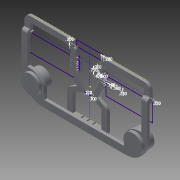
# Autodesk Inventor part: alignment_tool
Saved by Autodesk Inventor 2015 SP1 (Build 190203100, 203)
## iProperties
Created: 2015-09-17
Part Number: alignment_tool
Material: Generic
Document SubType Name: Modeling
Designer: tankadmin
Density: 1 g/cm^3
Appearance: Default
Author: tankadmin
Autodesk Inventor part; units mm, degrees
ref_plane "YZ Plane" through (0, 0, 0) normal (1, 0, 0) x (0, 1, 0)
ref_plane "XZ Plane" through (0, 0, 0) normal (0, 1, 0) x (-1, 0, 0)
ref_plane "XY Plane" through (0, 0, 0) normal (0, 0, 1) x (1, 0, 0)
sketch "Sketch1" plane through (0, 0, 0) normal (0, 0, 1) x (1, 0, 0)
  line L0 (-44.45, -76.2) -> (44.45, -76.2)
  line L1 (44.45, -76.2) -> (44.45, -19.05)
  line L2 (44.45, -19.05) -> (22.614, -6.964)
  line L3 (22.614, -6.964) -> (37.9893, 20.8148)
  line L4 (37.9893, 20.8148) -> (75.5958, 0)
  line L5 (75.5958, 0) -> (139.7, 0)
  line L6 (139.7, 0) -> (139.7, 76.2)
  line L7 (139.7, 76.2) -> (-139.7, 76.2)
  line L8 (-139.7, 76.2) -> (-139.7, 0)
  line L9 (-139.7, 0) -> (-75.5958, 0)
  line L10 (-75.5958, 0) -> (-37.9893, 20.8148)
  line L11 (-37.9893, 20.8148) -> (-22.614, -6.964)
  line L12 (-22.614, -6.964) -> (-44.45, -19.05)
  line L13 (-44.45, -19.05) -> (-44.45, -76.2)
  line L14 (0, -76.2) -> (0, 76.2) construction
  line L15 (-127, 63.5) -> (127, 63.5)
  line L16 (127, 63.5) -> (127, 12.7)
  line L17 (127, 12.7) -> (73.6309, 12.7)
  line L18 (73.6309, 12.7) -> (34.0201, 34.6241)
  line L19 (34.0201, 34.6241) -> (8.8047, -10.9331)
  line L20 (8.8047, -10.9331) -> (31.75, -23.6331)
  line L21 (31.75, -23.6331) -> (31.75, -63.5)
  line L22 (31.75, -63.5) -> (-31.75, -63.5)
  line L23 (-31.75, -63.5) -> (-31.75, -23.6331)
  line L24 (-31.75, -23.6331) -> (-8.8047, -10.9331)
  line L25 (-8.8047, -10.9331) -> (-34.0201, 34.6241)
  line L26 (-34.0201, 34.6241) -> (-73.6309, 12.7)
  line L27 (-73.6309, 12.7) -> (-127, 12.7)
  line L28 (-127, 12.7) -> (-127, 63.5)
  line L29 (139.7, 38.1) -> (-139.7, 38.1) construction
  line L30 (139.7, 19.05) -> (-139.7, 19.05) construction
  point P0 (0, 0)
  point P1 (0, 0)
  point P2 (0, 19.05)
  point P3 (25.4, 19.05)
  point P4 (-25.4, 19.05)
  dimension "d2" = 88.9
  dimension "d4" = 279.4
  dimension "d8" = 76.2
  dimension "d10" = 12.7
  dimension "d11" = 10.16
  dimension "d12" = 10.16
  dimension "d13" = 10.16
  dimension "d14" = 12.7
  dimension "d15" = 10.16
  dimension "d16" = 10.16
  dimension "d17" = 10.16
  dimension "d18" = 12.7
  dimension "d19" = 12.7
  dimension "d97" = 19.05
  dimension "d98" = 25.4
  dimension "d99" = 31.75
  dimension "d100" = 25.4
  dimension "d101" = 31.75
  dimension "d102" = 12.7
  dimension "d151" = 31.75
  dimension "d152" = 57.15
  dimension "d153" = 76.2
  constraints: 62 end point, 17 perpendicular, 8 point on line, 6 midpoint, 2 equal length, 1 coincident, 1 horizontal, 4 other
  measures "d2" distance between parallel lines of L1 L13
  measures "d4" distance between parallel lines of L6 L8
  measures "d8" distance between parallel lines of L0 L9
  measures "d10" distance between parallel lines of L22 L0
  measures "d11" distance between parallel lines of L24 L12
  measures "d12" distance between parallel lines of L25 L11
  measures "d13" distance between parallel lines of L10 L26
  measures "d14" distance between parallel lines of L9 L27
  measures "d15" distance between parallel lines of L2 L20
  measures "d16" distance between parallel lines of L3 L19
  measures "d17" distance between parallel lines of L4 L18
  measures "d18" distance between parallel lines of L5 L17
  measures "d19" distance between parallel lines of L6 L16
  measures "d97" distance between parallel lines of L30 L29
  measures "d98" distance of point (0, 19.05) point (25.4, 19.05)
  measures "d99" distance between parallel lines of L2 L4
  measures "d100" distance of point (-25.4, 19.05) point (0, 19.05)
  measures "d101" distance between parallel lines of L10 L12
  measures "d102" vertical distance of L19.end L20.end
  measures "d151" distance from line of L17 L1.end
  measures "d152" distance from line of L1.end L29
  measures "d153" distance between parallel lines of L5 L7
extrude "Extrusion1" add sketch "Sketch1" along normal blind 6.35
sketch "Sketch2" plane through (0, 0, 6.35) normal (0, 0, 1) x (1, 0, 0)
  line L0 (31.75, -63.5) -> (-31.75, -63.5) construction
  line L1 (139.7, 50.8) -> (139.7, -78.74)
  line L2 (139.7, -78.74) -> (-139.7, -78.74)
  line L3 (-139.7, -78.74) -> (-139.7, 50.8)
  circle A0 centre (-114.3, -43.18) radius 13.081
  line L4 (0, -78.74) -> (0, 75.1889) construction
  line L5 (-139.7, 45.72) -> (139.7, 45.72) construction
  circle A1 centre (114.3, -43.18) radius 13.081
  line L6 (-127, -17.78) -> (-127, 50.8)
  line L7 (-127, 50.8) -> (-139.7, 50.8)
  line L8 (127, -17.78) -> (127, 50.8)
  line L9 (139.7, 76.2) -> (-139.7, 76.2) construction
  line L10 (139.7, 50.8) -> (127, 50.8)
  line L11 (-127, -17.78) -> (-88.9, -17.78)
  line L12 (88.9, -17.78) -> (127, -17.78)
  line L13 (-88.9, -63.5) -> (-88.9, -17.78)
  line L14 (-88.9, -63.5) -> (88.9, -63.5)
  line L15 (88.9, -63.5) -> (88.9, -17.78)
  line L16 (-127, 12.7) -> (-127, 63.5) projected
  line L17 (127, 63.5) -> (127, 12.7) projected
  line L18 (-127, 63.5) -> (127, 63.5) construction
  line L19 (-139.7, 0) -> (-75.5958, 0) projected
  point P0 (0, 0)
  dimension "d24" = 15.24
  dimension "d25" = 26.162
  dimension "d28" = 114.3
  dimension "d34" = 88.9
  dimension "d119" = 12.7
  dimension "d120" = 12.7
  dimension "d121" = 25.4
  dimension "d142" = 25.4
  dimension "d150" = 5.08
  dimension "d155" = 43.18
  constraints: 28 end point, 5 collinear, 5 perpendicular, 2 centre point, 2 parallel, 2 point on line, 1 horizontal, 1 midpoint, 1 symmetric about line, 1 vertical, 2 other
  measures "d24" distance between parallel lines of L2 L0
  measures "d25" diameter of A0
  measures "d28" distance from line of A0.centre L4
  measures "d34" distance from line of A0.centre L5
  measures "d119" distance between parallel lines of L3 L6
  measures "d120" distance between parallel lines of L1 L8
  measures "d121" distance from line of L13 A0.centre
  measures "d142" distance from line of A0.centre L11
  measures "d150" distance between parallel lines of L5 L7
  measures "d155" distance from line of A0.centre L19
extrude "Extrusion2" add sketch "Sketch2" along normal blind 6.35
sketch "Sketch3" plane through (0, 0, 12.7) normal (0, 0, 1) x (1, 0, 0)
  circle A0 centre (-114.3, -43.18) radius 13.081 construction
  circle A1 centre (114.3, -43.18) radius 13.081 construction
  circle A2 centre (-114.3, -43.18) radius 20.701
  circle A3 centre (114.3, -43.18) radius 20.701
  point P0 (0, 0)
  dimension "d37" = 7.62
  dimension "d38" = 7.62
  constraints: 2 centre point, 2 coincident
  measures "d37" radial gap between concentric circles of A2 A0
  measures "d38" radial gap between concentric circles of A3 A1
extrude "Extrusion3" add sketch "Sketch3" along normal blind 6.35
sketch "Sketch4" plane through (0, 0, 6.35) normal (0, 0, -1) x (-1, 0, 0)
  circle A0 centre (-114.3, -43.18) radius 13.081 construction
  line L0 (-139.7, -78.74) -> (-139.7, -78.74) construction
  line L1 (44.45, -76.2) -> (-44.45, -76.2) construction
  line L2 (139.7, -78.74) -> (-139.7, -78.74) construction
  line L3 (-139.7, 0) -> (-139.7, 76.2) construction
  line L4 (0, -78.74) -> (0, 89.4584) construction
  line L5 (152.4, 45.72) -> (-152.4, 45.72) construction
  line L6 (-0.635, -76.2) -> (0.635, -76.2)
  line L7 (0.635, -76.2) -> (0.635, -78.74)
  line L8 (0.635, -78.74) -> (-0.635, -78.74)
  line L9 (-0.635, -78.74) -> (-0.635, -76.2)
  line L10 (-73.6309, 12.7) -> (-34.0201, 34.6241) construction
  line L11 (-31.75, -23.6331) -> (-8.8047, -10.9331) construction
  line L12 (73.6309, 12.7) -> (34.0201, 34.6241) construction
  line L13 (38.4647, 32.1641) -> (13.2493, -13.3932) construction
  line L14 (8.8047, -10.9331) -> (34.0201, 34.6241) construction
  line L15 (22.614, -6.964) -> (37.9893, 20.8148) construction
  circle A1 centre (-114.3, -43.18) radius 13.081 projected
  circle A2 centre (114.3, -43.18) radius 13.081 projected
  line L16 (-127, 50.8) -> (-127, 12.7) projected
  line L17 (-75.5958, 0) -> (-127, 0) projected
  line L18 (-37.9893, 20.8148) -> (-75.5958, 0) projected
  line L19 (-22.614, -6.964) -> (-37.9893, 20.8148) projected
  line L20 (-44.45, -19.05) -> (-22.614, -6.964) projected
  line L21 (-44.45, -63.5) -> (-44.45, -19.05) projected
  line L22 (-88.9, -63.5) -> (-44.45, -63.5) projected
  line L23 (-88.9, -17.78) -> (-88.9, -63.5) projected
  line L24 (-127, 0) -> (-139.7, 0) projected
  line L25 (-139.7, -78.74) -> (-139.7, 0) projected
  line L26 (139.7, -78.74) -> (-139.7, -78.74) projected
  line L27 (139.7, 0) -> (139.7, -78.74) projected
  line L28 (139.7, 0) -> (127, 0) projected
  line L29 (127, 0) -> (75.5958, 0) projected
  line L30 (75.5958, 0) -> (37.9893, 20.8148) projected
  line L31 (37.9893, 20.8148) -> (22.614, -6.964) projected
  line L32 (22.614, -6.964) -> (44.45, -19.05) projected
  line L33 (44.45, -19.05) -> (44.45, -63.5) projected
  line L34 (44.45, -63.5) -> (44.45, -76.2) projected
  line L35 (44.45, -76.2) -> (-44.45, -76.2) projected
  line L36 (-44.45, -76.2) -> (-44.45, -63.5) projected
  line L37 (-44.45, -63.5) -> (-31.75, -63.5) projected
  line L38 (-31.75, -23.6331) -> (-31.75, -63.5) projected
  line L39 (-8.8047, -10.9331) -> (-31.75, -23.6331) projected
  line L40 (-34.0201, 34.6241) -> (-8.8047, -10.9331) projected
  line L41 (-73.6309, 12.7) -> (-34.0201, 34.6241) projected
  line L42 (-127, 12.7) -> (-73.6309, 12.7) projected
  line L43 (127, 63.5) -> (-127, 63.5) projected
  line L44 (88.9, -63.5) -> (88.9, -17.78) projected
  line L45 (44.45, -63.5) -> (88.9, -63.5) projected
  line L46 (31.75, -63.5) -> (44.45, -63.5) projected
  line L47 (31.75, -63.5) -> (31.75, -23.6331) projected
  line L48 (31.75, -23.6331) -> (8.8047, -10.9331) projected
  line L49 (8.8047, -10.9331) -> (34.0201, 34.6241) projected
  line L50 (34.0201, 34.6241) -> (73.6309, 12.7) projected
  line L51 (73.6309, 12.7) -> (127, 12.7) projected
  line L52 (-31.75, -63.5) -> (31.75, -63.5) projected
  line L53 (127, 12.7) -> (127, 50.8) projected
  line L54 (-127, -17.78) -> (-88.9, -17.78) projected
  line L55 (-127, 0) -> (-127, -17.78) projected
  line L56 (127, 0) -> (127, 12.7) projected
  line L57 (127, -17.78) -> (127, 0) projected
  line L58 (88.9, -17.78) -> (127, -17.78) projected
  line L59 (-88.9, -63.5) -> (88.9, -63.5) projected
  line L60 (0.635, -63.5) -> (-0.635, -63.5)
  line L61 (-0.635, -63.5) -> (-0.635, -60.96)
  line L62 (-0.635, -60.96) -> (0.635, -60.96)
  line L63 (0.635, -60.96) -> (0.635, -63.5)
  line L64 (127, 50.8) -> (139.7, 50.8) projected
  line L65 (139.7, 76.2) -> (139.7, 50.8) construction
  line L66 (-139.7, 76.2) -> (139.7, 76.2) projected
  line L67 (-139.7, 50.8) -> (-139.7, 76.2) projected
  line L68 (-139.7, 50.8) -> (-127, 50.8) projected
  line L69 (-127, 12.7) -> (-127, 0) projected
  line L70 (127, 50.8) -> (127, 63.5) projected
  line L71 (-127, 63.5) -> (-127, 50.8) projected
  line L72 (124.46, 46.355) -> (127, 46.355)
  line L73 (127, 46.355) -> (127, 45.085)
  line L74 (127, 45.085) -> (124.46, 45.085)
  line L75 (124.46, 45.085) -> (124.46, 46.355)
  line L76 (139.7, 63.5) -> (139.7, 12.7) construction
  line L77 (-124.46, 46.355) -> (-127, 46.355)
  line L78 (-127, 46.355) -> (-127, 45.085)
  line L79 (-127, 45.085) -> (-124.46, 45.085)
  line L80 (-124.46, 45.085) -> (-124.46, 46.355)
  line L81 (-139.7, 0) -> (-139.7, 50.8) projected
  line L82 (139.7, 50.8) -> (139.7, 0) projected
  line L83 (12.065, -76.2) -> (13.335, -76.2)
  line L84 (13.335, -76.2) -> (13.335, -78.74)
  line L85 (13.335, -78.74) -> (12.065, -78.74)
  line L86 (12.065, -78.74) -> (12.065, -76.2)
  line L87 (13.335, -63.5) -> (12.065, -63.5)
  line L88 (12.065, -63.5) -> (12.065, -60.96)
  line L89 (12.065, -60.96) -> (13.335, -60.96)
  line L90 (13.335, -60.96) -> (13.335, -63.5)
  line L91 (-13.335, -76.2) -> (-12.065, -76.2)
  line L92 (-12.065, -76.2) -> (-12.065, -78.74)
  line L93 (-12.065, -78.74) -> (-13.335, -78.74)
  line L94 (-13.335, -78.74) -> (-13.335, -76.2)
  line L95 (-12.065, -63.5) -> (-13.335, -63.5)
  line L96 (-13.335, -63.5) -> (-13.335, -60.96)
  line L97 (-13.335, -60.96) -> (-12.065, -60.96)
  line L98 (-12.065, -60.96) -> (-12.065, -63.5)
  line L99 (-0.635, -76.2) -> (0.635, -76.2)
  line L100 (0.635, -76.2) -> (0.635, -78.74)
  line L101 (0.635, -78.74) -> (-0.635, -78.74)
  line L102 (-0.635, -78.74) -> (-0.635, -76.2)
  line L103 (0.635, -63.5) -> (-0.635, -63.5)
  line L104 (-0.635, -63.5) -> (-0.635, -60.96)
  line L105 (-0.635, -60.96) -> (0.635, -60.96)
  line L106 (0.635, -60.96) -> (0.635, -63.5)
  point P0 (0, 0)
  point P1 (0, -78.74)
  point P2 (124.46, 45.72)
  point P3 (-124.46, 45.72)
  point P4 (12.7, -78.74)
  point P5 (12.7, -78.74)
  point P6 (-12.7, -78.74)
  point P7 (-12.7, -78.74)
  point P8 (0, -78.74)
  dimension "d67" = 1.27
  dimension "d68" = 2.54
  dimension "d124" = 88.9
  dimension "d147" = 2.54
  dimension "d156" = 2.54
  dimension "d157" = 1.27
  dimension "d165" = 12.7
  dimension "d168" = 12.7
  constraints: 92 end point, 10 symmetric about line, 6 horizontal, 6 parallel, 5 point on line, 4 perpendicular, 3 collinear, 3 midpoint, 55 other
  measures "d67" distance between parallel lines of L9 L7
  measures "d68" distance between parallel lines of L8 L1
  measures "d124" distance from line of A0.centre L5
  measures "d147" distance between parallel lines of L52 L62
  measures "d156" distance between parallel lines of L73 L75
  measures "d157" distance between parallel lines of L74 L72
  measures "d165" distance of L61.end L89.start
  measures "d168" distance of L61.end L97.start
sketch "Sketch5" plane through (0, 0, 6.35) normal (0, 0, -1) x (-1, 0, 0)
  circle A0 centre (-114.3, -43.18) radius 13.081 projected
  circle A1 centre (-114.3, -43.18) radius 20.701 projected
  circle A2 centre (114.3, -43.18) radius 13.081 projected
  circle A3 centre (114.3, -43.18) radius 20.701 projected
  point P0 (0, 0)
extrude "Extrusion5" add sketch "Sketch5" along normal blind 15.24
fillet "Fillet1" radius 12.7 10 edges at (139.7, 76.2, 3.175) (-139.7, 76.2, 3.175) (139.7, 0, 3.175) (-139.7, 0, 3.175) (44.45, -76.2, 3.175) (-44.45, -76.2, 3.175) (-75.5958, 0, 3.175) (-44.45, -19.05, 3.175) (44.45, -19.05, 3.175) (75.5958, 0, 3.175)
sketch "Sketch6" plane through (0, 0, 0) normal (0, 0, -1) x (-1, 0, 0)
  point P0 (0, 0)
extrude "Extrusion6" add sketch "Sketch4" along normal blind 6.35 contours L6 L7 L8 L9 | L92 L26 L94 L35 | L35 L84 L26 L86 | L96 L97 L98 L52 | L52 L88 L89 L90 | L16 L77 L80 L79 | L61 L62 L63 L52 | L74 L75 L72 L53
sketch "Sketch7" plane through (0, 0, 0) normal (0, 0, -1) x (-1, 0, 0)
  line L0 (-127, 76.2) -> (127, 76.2) construction
  line L1 (0, 76.2) -> (0, -78.74) construction
  line L2 (139.7, -78.74) -> (-139.7, -78.74) construction
  line L3 (-8.8047, -10.9331) -> (-34.0201, 34.6241) construction
  line L4 (-31.75, -23.6331) -> (-8.8047, -10.9331) construction
  line L5 (-35.56, 63.5) -> (-25.4, 63.5)
  line L6 (-25.4, 63.5) -> (-25.4, 19.05)
  line L7 (-35.56, 33.7718) -> (-35.56, 63.5)
  line L8 (-25.4, 19.05) -> (-35.56, 33.7718)
  line L9 (-34.0201, 34.6241) -> (-73.6309, 12.7) construction
  line L10 (35.56, 63.5) -> (25.4, 63.5)
  line L11 (25.4, 63.5) -> (25.4, 19.05)
  line L12 (35.56, 33.7718) -> (35.56, 63.5)
  line L13 (25.4, 19.05) -> (35.56, 33.7718)
  line L14 (-127, 63.5) -> (127, 63.5) construction
  point P0 (0, 0)
  dimension "d106" = 10.16
  dimension "d158" = 25.4
  constraints: 18 end point, 4 symmetric about line, 2 midpoint, 2 point on line, 1 collinear, 1 perpendicular
  measures "d106" distance between parallel lines of L7 L6
  measures "d158" distance between parallel lines of L1 L6
extrude "Extrusion11" add sketch "Sketch7" against normal blind 6.35
sketch "Sketch8" plane through (0, 0, 0) normal (0, 0, -1) x (-1, 0, 0)
  line L0 (-127, 76.2) -> (127, 76.2) construction
  line L1 (0, 76.2) -> (0, -63.5) construction
  line L2 (31.75, -63.5) -> (-31.75, -63.5) construction
  line L3 (-30.48, 63.5) -> (-30.48, 17.7379)
  line L4 (-30.48, 17.7379) -> (-11.7992, -16.0131)
  line L5 (-11.7992, -16.0131) -> (11.7992, -16.0131)
  line L6 (11.7992, -16.0131) -> (30.48, 17.7379)
  line L7 (30.48, 17.7379) -> (30.48, 63.5)
  line L8 (30.48, 63.5) -> (-30.48, 63.5)
  line L9 (-8.8047, -10.9331) -> (-34.0201, 34.6241) construction
  line L10 (-25.4, 63.5) -> (-25.4, 19.05) construction
  line L11 (-25.4, 63.5) -> (25.4, 63.5) projected
  line L12 (-30.48, 76.2) -> (30.48, 76.2)
  line L13 (30.48, 76.2) -> (30.48, 63.5)
  line L14 (30.48, 63.5) -> (-30.48, 63.5)
  line L15 (-30.48, 63.5) -> (-30.48, 76.2)
  line L16 (-38.1, 27.305) -> (-22.86, 27.305)
  line L17 (-22.86, 27.305) -> (-22.86, 26.035)
  line L18 (-22.86, 26.035) -> (-38.1, 26.035)
  line L19 (-38.1, 26.035) -> (-38.1, 27.305)
  line L20 (-38.1, 32.0675) -> (-22.86, 32.0675)
  line L21 (-22.86, 32.0675) -> (-22.86, 30.7975)
  line L22 (-22.86, 30.7975) -> (-38.1, 30.7975)
  line L23 (-38.1, 30.7975) -> (-38.1, 32.0675)
  line L24 (-38.1, 35.2425) -> (-22.86, 35.2425)
  line L25 (-22.86, 35.2425) -> (-22.86, 33.9725)
  line L26 (-22.86, 33.9725) -> (-38.1, 33.9725)
  line L27 (-38.1, 33.9725) -> (-38.1, 35.2425)
  line L28 (-38.1, 38.4175) -> (-22.86, 38.4175)
  line L29 (-22.86, 38.4175) -> (-22.86, 37.1475)
  line L30 (-22.86, 37.1475) -> (-38.1, 37.1475)
  line L31 (-38.1, 37.1475) -> (-38.1, 38.4175)
  line L32 (-38.1, 22.5425) -> (-22.86, 22.5425)
  line L33 (-22.86, 22.5425) -> (-22.86, 21.2725)
  line L34 (-22.86, 21.2725) -> (-38.1, 21.2725)
  line L35 (-38.1, 21.2725) -> (-38.1, 22.5425)
  line L36 (38.1, 27.305) -> (22.86, 27.305)
  line L37 (22.86, 27.305) -> (22.86, 26.035)
  line L38 (22.86, 26.035) -> (38.1, 26.035)
  line L39 (38.1, 26.035) -> (38.1, 27.305)
  line L40 (38.1, 32.0675) -> (22.86, 32.0675)
  line L41 (22.86, 32.0675) -> (22.86, 30.7975)
  line L42 (22.86, 30.7975) -> (38.1, 30.7975)
  line L43 (38.1, 30.7975) -> (38.1, 32.0675)
  line L44 (38.1, 35.2425) -> (22.86, 35.2425)
  line L45 (22.86, 35.2425) -> (22.86, 33.9725)
  line L46 (22.86, 33.9725) -> (38.1, 33.9725)
  line L47 (38.1, 33.9725) -> (38.1, 35.2425)
  line L48 (38.1, 38.4175) -> (22.86, 38.4175)
  line L49 (22.86, 38.4175) -> (22.86, 37.1475)
  line L50 (22.86, 37.1475) -> (38.1, 37.1475)
  line L51 (38.1, 37.1475) -> (38.1, 38.4175)
  line L52 (38.1, 22.5425) -> (22.86, 22.5425)
  line L53 (22.86, 22.5425) -> (22.86, 21.2725)
  line L54 (22.86, 21.2725) -> (38.1, 21.2725)
  line L55 (38.1, 21.2725) -> (38.1, 22.5425)
  line L56 (-38.1, 46.355) -> (-22.86, 46.355)
  line L57 (-22.86, 46.355) -> (-22.86, 45.085)
  line L58 (-22.86, 45.085) -> (-38.1, 45.085)
  line L59 (-38.1, 45.085) -> (-38.1, 46.355)
  line L60 (38.1, 46.355) -> (22.86, 46.355)
  line L61 (22.86, 46.355) -> (22.86, 45.085)
  line L62 (22.86, 45.085) -> (38.1, 45.085)
  line L63 (38.1, 45.085) -> (38.1, 46.355)
  line L64 (35.56, 33.7718) -> (35.56, 63.5) construction
  line L65 (139.7, 0) -> (35.56, 0)
  line L66 (35.56, 0) -> (35.56, 39.37)
  line L67 (139.7, 39.37) -> (139.7, 0)
  line L68 (127, 0) -> (78.876, 0) projected
  line L69 (-139.7, 0) -> (-35.56, 0)
  line L70 (-35.56, 0) -> (-35.56, 39.37)
  line L71 (-139.7, 39.37) -> (-139.7, 0)
  line L72 (-127, 0) -> (-78.876, 0)
  line L73 (-139.7, 39.37) -> (-35.56, 39.37)
  line L74 (139.7, 39.37) -> (35.56, 39.37)
  line L75 (127, 46.355) -> (124.46, 46.355) construction
  line L76 (124.46, 45.085) -> (127, 45.085) construction
  line L77 (-127, 45.085) -> (-124.46, 45.085) construction
  line L78 (-124.46, 46.355) -> (-127, 46.355) construction
  line L79 (-124.46, 45.72) -> (124.46, 45.72) construction
  line L80 (139.7, -78.74) -> (139.7, 12.7) construction
  line L81 (-124.46, 45.085) -> (-124.46, 46.355) construction
  line L82 (124.46, 46.355) -> (124.46, 45.085) construction
  point P0 (0, 0)
  point P1 (-30.48, 26.035)
  point P2 (-22.86, 26.67)
  point P3 (-22.86, 31.4325)
  point P4 (-22.86, 34.6075)
  point P5 (-22.86, 37.7825)
  point P6 (-22.86, 21.9075)
  point P7 (-30.48, 21.2725)
  point P8 (-30.48, 30.7975)
  point P9 (-30.48, 33.9725)
  point P10 (-30.48, 37.1475)
  point P11 (30.48, 26.035)
  point P12 (22.86, 26.67)
  point P13 (22.86, 31.4325)
  point P14 (22.86, 34.6075)
  point P15 (22.86, 37.7825)
  point P16 (22.86, 21.9075)
  point P17 (30.48, 30.7975)
  point P18 (30.48, 33.9725)
  point P19 (30.48, 37.1475)
  point P20 (-22.86, 45.72)
  point P21 (-30.48, 45.085)
  point P22 (22.86, 45.72)
  point P23 (30.48, 45.085)
  dimension "d105" = 5.08
  dimension "d109" = 5.08
  dimension "d110" = 5.08
  dimension "d111" = 0
  dimension "d133" = 1.27
  dimension "d134" = 15.24
  dimension "d136" = 4.7625
  dimension "d137" = 4.7625
  dimension "d138" = 3.175
  dimension "d139" = 3.175
  dimension "d159" = 0
  dimension "d160" = 19.05
  dimension "d162" = 6.35
  constraints: 138 end point, 41 symmetric about line, 17 parallel, 16 midpoint, 10 equal length, 10 perpendicular, 9 horizontal, 7 point on line, 6 collinear, 1 vertical, 2 other
  measures "d105" distance between parallel lines of L9 L4
  measures "d109" distance between parallel lines of L10 L3
  measures "d110" distance from line of L5 L9.start
  measures "d111" distance between parallel lines of L11 L8
  measures "d133" distance between parallel lines of L18 L16
  measures "d134" distance between parallel lines of L17 L19
  measures "d136" distance of point (-22.86, 31.433) point (-22.86, 26.67)
  measures "d137" distance of point (-22.86, 21.908) point (-22.86, 26.67)
  measures "d138" distance of point (-22.86, 34.608) point (-22.86, 31.433)
  measures "d139" distance of point (-22.86, 37.783) point (-22.86, 34.608)
  measures "d159" distance from line of L79 point (-22.86, 45.72)
  measures "d160" distance from line of point (-22.86, 26.67) L79
  measures "d162" distance between parallel lines of L73 L79
extrude "Extrusion15" cut sketch "Sketch8" against normal blind 6.35 contours L70 L30 L31 L28 | L28 L31 L30 L70 L24 L27 L26 L20 L23 L22 L16 L19 L18 L32 L35 L34 L69 L71 L73 | L70 L26 L27 L24 | L66 L74 L67 L65 L54 L55 L52 L38 L39 L36 L42 L43 L40 L46 L47 L44 L50 L51 L48 | L48 L51 L50 L66 | L70 L22 L23 L20 | L44 L47 L46 L66 | L70 L18 L19 L16 | L34 L35 L32 L70 | L40 L43 L42 L66 | L36 L39 L38 L66 | L66 L52 L55 L54
extrude "Extrusion14" add sketch "Sketch8" against normal blind 6.35 contours L56 L57 L58 L3 | L3 L58 L59 L56 | L28 L29 L30 L3 | L3 L30 L70 L28 | L70 L30 L31 L28 | L60 L63 L62 L7 | L7 L62 L61 L60 | L24 L25 L26 L3 | L3 L26 L70 L24 | L70 L26 L27 L24 | L48 L66 L50 L7 | L7 L50 L49 L48 | L20 L21 L22 L3 | L3 L22 L70 L20 | L48 L51 L50 L66 | L70 L22 L23 L20 | L44 L66 L46 L7 | L7 L46 L45 L44 | L16 L17 L18 L3 | L3 L18 L70 L16 | L44 L47 L46 L66 | L70 L18 L19 L16 | L40 L66 L42 L7 | L7 L42 L41 L40 | L32 L33 L34 L3 | L3 L34 L70 L32 | L34 L35 L32 L70 | L40 L43 L42 L66 | L36 L66 L38 L7 | L7 L38 L37 L36 | L36 L39 L38 L66 | L52 L66 L54 L7 | L7 L54 L53 L52 | L66 L52 L55 L54
extrude "Extrusion12" cut sketch "Sketch8" against normal through all contours L15 L12 L13 L8
extrude "Extrusion13" cut sketch "Sketch8" against normal blind 1.27 contours L8 L7 L60 L61 L62 L48 L49 L50 L44 L45 L46 L40 L41 L42 L36 L37 L38 L52 L53 L54 L6 L5 L4 L3 L34 L33 L32 L18 L17 L16 L22 L21 L20 L26 L25 L24 L30 L29 L28 L58 L57 L56 | L56 L57 L58 L3 | L28 L29 L30 L3 | L7 L62 L61 L60 | L24 L25 L26 L3 | L7 L50 L49 L48 | L20 L21 L22 L3 | L7 L46 L45 L44 | L16 L17 L18 L3 | L7 L42 L41 L40 | L32 L33 L34 L3 | L7 L38 L37 L36 | L7 L54 L53 L52
fillet "Fillet4" radius 12.7 2 edges at (35.56, 63.5, 3.175) (-35.56, 63.5, 3.175)
fillet "Fillet5" radius 5.08 2 edges at (-25.4, 63.5, 3.81) (25.4, 63.5, 3.81)
fillet "Fillet7" radius 38.1 2 edges at (88.9, -17.78, 9.525) (-88.9, -17.78, 9.525) curvature continuous yes
fillet "Fillet8" radius 53.34 2 edges at (139.7, -78.74, 9.525) (-139.7, -78.74, 9.525) curvature continuous yes
fillet "Fillet10" radius 0.635 64 edges at (22.86, 21.2725, 3.81) (22.86, 22.5425, 3.81) (22.86, 26.035, 3.81) (22.86, 27.305, 3.81) (22.86, 30.7975, 3.81) (22.86, 32.0675, 3.81) (22.86, 33.9725, 3.81) (22.86, 35.2425, 3.81) (22.86, 37.1475, 3.81) (22.86, 38.4175, 3.81) (22.86, 45.085, 3.81) (22.86, 46.355, 3.81) (-22.86, 46.355, 3.81) (-22.86, 45.085, 3.81) (-22.86, 38.4175, 3.81) (-22.86, 37.1475, 3.81) (-22.86, 35.2425, 3.81) (-22.86, 33.9725, 3.81) (-22.86, 32.0675, 3.81) (-22.86, 30.7975, 3.81) (-22.86, 27.305, 3.81) (-22.86, 26.035, 3.81) (-22.86, 22.5425, 3.81) (-22.86, 21.2725, 3.81) (-38.1, 46.355, 3.175) (-38.1, 45.085, 3.175) (-38.1, 27.305, 3.175) (-38.1, 26.035, 3.175) (-38.1, 22.5425, 3.175) (-38.1, 21.2725, 3.175) (38.1, 46.355, 3.175) (38.1, 45.085, 3.175) (38.1, 27.305, 3.175) (38.1, 26.035, 3.175) (38.1, 22.5425, 3.175) (38.1, 21.2725, 3.175) (0.635, -60.96, 3.175) (-0.635, -60.96, 3.175) (-0.635, -78.74, 3.175) (0.635, -78.74, 3.175) (38.1, 38.4175, 3.175) (38.1, 37.1475, 3.175) (38.1, 35.2425, 3.175) (38.1, 33.9725, 3.175) (38.1, 32.0675, 3.175) (38.1, 30.7975, 3.175) (-38.1, 38.4175, 3.175) (-38.1, 37.1475, 3.175) (-38.1, 35.2425, 3.175) (-38.1, 33.9725, 3.175) (-38.1, 32.0675, 3.175) (-38.1, 30.7975, 3.175) (124.46, 46.355, 3.175) (124.46, 45.085, 3.175) (-124.46, 46.355, 3.175) (-124.46, 45.085, 3.175) (12.065, -60.96, 3.175) (13.335, -60.96, 3.175) (-12.065, -60.96, 3.175) (-13.335, -60.96, 3.175) (-13.335, -78.74, 3.175) (-12.065, -78.74, 3.175) (12.065, -78.74, 3.175) (13.335, -78.74, 3.175)
fillet "Fillet11" radius 6.35 4 edges at (133.35, 50.8, 12.7) (133.35, 39.37, 0) (-133.35, 50.8, 12.7) (-133.35, 39.37, 0)
equation "\"d11\" = d13"
equation "\"d12\" = d13"
equation "\"d14\" = d10"
equation "\"d15\" = d13"
equation "\"d16\" = d13"
equation "\"d17\" = d13"
equation "\"d18\" = d10"
equation "\"d19\" = d10"
equation "\"d38\" = d37"
equation "\"d67\" = d51"
equation "\"d68\" = d52"
equation "\"d51\" = 1.27"
equation "\"d52\" = 2.54"
body "Solid1"
